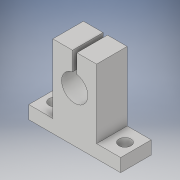
# Autodesk Inventor part: SK12
Saved by Autodesk Inventor 2019 (Build 230136000, 136)
## iProperties
Created: 2020-01-19
Part Number: SK12
Material: Generic
Document SubType Name: Modeling
Designer: Dell-T1700
Density: 1 g/cm^3
Appearance: Default
Author: Dell-T1700
Autodesk Inventor part; units mm, degrees
ref_plane "YZ Plane" through (0, 0, 0) normal (1, 0, 0) x (0, 1, 0)
ref_plane "XZ Plane" through (0, 0, 0) normal (0, 1, 0) x (-1, 0, 0)
ref_plane "XY Plane" through (0, 0, 0) normal (0, 0, 1) x (1, 0, 0)
sketch "Sketch1" plane through (0, 0, 0) normal (0, 0, 1) x (1, 0, 0)
  arc A0 (-1, 5.9161) -> (1, 5.9161) centre (0, 0) ccw
  line L0 (-21, -23) -> (21, -23)
  line L1 (-21, -23) -> (-21, -17)
  line L2 (21, -23) -> (21, -17)
  line L3 (-10, 14.5) -> (-10, -17)
  line L4 (-10, -17) -> (-21, -17)
  line L5 (-10, 14.5) -> (-1, 14.5)
  line L6 (10, 14.5) -> (1, 14.5)
  line L7 (1, 14.5) -> (1, 5.9161)
  line L8 (-1, 14.5) -> (-1, 5.9161)
  line L9 (10, 14.5) -> (10, -17)
  line L10 (10, -17) -> (21, -17)
  dimension "d0" = 12
  dimension "d1" = 23
  dimension "d2" = 42
  dimension "d3" = 21
  dimension "d4" = 6
  dimension "d7" = 9
  dimension "d8" = 9
  dimension "d10" = 37.5
  dimension "d11" = 37.5
  dimension "d14" = 10
  dimension "d15" = 31.5
  dimension "d16" = 6
  dimension "d17" = 10
  constraints: 22 end point, 4 vertical, 3 horizontal, 3 perpendicular, 2 point on circle, 1 centre point, 1 coincident
  measures "d0" diameter of A0
  measures "d1" distance from line of L0 point (0, 0)
  measures "d2" distance of L0.start L0.end
  measures "d3" horizontal distance of L0.end point (0, 0)
  measures "d4" distance of L0.start L1.end
  measures "d7" distance of L3.start L5.end
  measures "d8" distance of L6.start L6.end
  measures "d10" distance between parallel lines of L0 L6
  measures "d11" distance between parallel lines of L0 L5
  measures "d14" distance from line of point (0, 0) L3
  measures "d15" distance of L3.start L3.end
  measures "d16" distance from line of L0 L2.end
  measures "d17" distance from line of point (0, 0) L9
extrude "Extrusion1" add sketch "Sketch1" along normal blind 14
sketch "Sketch2" plane through (10, -17, 0) normal (0, 1, 0) x (1, 0, 0)
  circle A0 centre (-26, -7) radius 2.75
  circle A1 centre (6, -7) radius 2.75
  line L0 (-10, 2.8) -> (-10, -16.8) projected
  line L1 (-20, -14) -> (-31, -14) projected
  point P0 (-10, 0)
  dimension "d20" = 5.5
  dimension "d21" = 5.5
  dimension "d22" = 32
  dimension "d23" = 16
  dimension "d24" = 7
  dimension "d25" = 16
  constraints: 2 centre point
  measures "d20" diameter of A0
  measures "d21" diameter of A1
  measures "d22" distance of A1.centre A0.centre
  measures "d23" distance from line of L0 A0.centre
  measures "d24" distance from line of L1 A0.centre
  measures "d25" distance from line of A1.centre L0
extrude "Extrusion2" cut sketch "Sketch2" against normal blind 14
body "Solid1"
